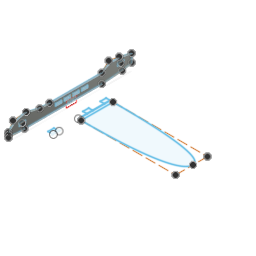
Plane v9 (Autodesk Fusion 360 design; units mm, degrees)
Autodesk Fusion 360 part; units mm, degrees
sketch "Body" plane through (0, 0, 0) normal (1, 0, 0) x (0, 0, -1)
  line L0 (-108.4233, 7.9987) -> (-100.7784, 21.612)
  line L1 (-100.7784, 21.612) -> (-77.9041, 23.072)
  spline S0 degree 2 poles (-108.4233, 7.9987) (-100.7784, 21.612) (-77.9041, 23.072) knots 0 0 0 1 1 1
  line L2 (-77.9041, 23.072) -> (-54.5916, 16.5393)
  line L3 (-54.5916, 16.5393) -> (-37.5103, 16.5393)
  spline S1 degree 2 poles (-77.9041, 23.072) (-54.5916, 16.5393) (-37.5103, 16.5393) knots 0 0 0 1 1 1
  line L4 (-37.5103, 16.5393) -> (52.5, 16.5392)
  line L5 (52.5, 16.5392) -> (64.5, 28.5)
  line L6 (64.5, 28.5) -> (82.5, 25.5)
  line L7 (82.5, 25.5) -> (104.0184, 19.9474)
  spline S2 degree 3 poles (52.5, 16.5392) (64.5, 28.5) (82.5, 25.5) (104.0184, 19.9474) knots 0 0 0 0 1 1 1 1
  line L8 (104.0184, 19.9474) -> (104.0184, 6)
  line L9 (104.0184, 6) -> (87.6259, 2.2265)
  line L10 (87.6259, 2.2265) -> (52.5, 0)
  spline S3 degree 2 poles (104.0184, 6) (87.6259, 2.2265) (52.5, 0) knots 0 0 0 1 1 1
  line L11 (52.5, 0) -> (-81.1435, 0.0002)
  line L12 (-108.4233, 7.9987) -> (-108.4233, 4.4987)
  line L13 (-108.4233, 4.4987) -> (-108.4233, -0.1059)
  line L14 (-108.4233, -0.1059) -> (-81.1435, 0.0002)
  spline S4 degree 2 poles (-108.4233, 4.4987) (-108.4233, -0.1059) (-81.1435, 0.0002) knots 0 0 0 1 1 1
  line L15 (0, 9) -> (2.5, 9) construction
  line L16 (2.5, 9) -> (2.5, 10.75) construction
  line L17 (2.5, 10.75) -> (12.5, 10.75)
  line L18 (12.5, 10.75) -> (12.5, 7.25)
  line L19 (12.5, 7.25) -> (2.5, 7.25)
  line L20 (2.5, 7.25) -> (2.5, 10.75)
  line L21 (12.5, 10.75) -> (17.5, 10.75) construction
  line L22 (17.5, 10.75) -> (27.5, 10.75)
  line L23 (27.5, 10.75) -> (27.5, 7.25)
  line L24 (27.5, 7.25) -> (17.5, 7.25)
  line L25 (17.5, 7.25) -> (17.5, 10.75)
  line L26 (0, 9) -> (-2.5, 9) construction
  line L27 (-2.5, 9) -> (-2.5, 10.75) construction
  line L28 (-2.5, 10.75) -> (-12.5, 10.75)
  line L29 (-12.5, 10.75) -> (-12.5, 7.25)
  line L30 (-12.5, 7.25) -> (-2.5, 7.25)
  line L31 (-2.5, 7.25) -> (-2.5, 10.75)
  line L32 (-12.5, 10.75) -> (-17.5, 10.75) construction
  line L33 (-17.5, 10.75) -> (-27.5, 10.75)
  line L34 (-27.5, 10.75) -> (-27.5, 7.25)
  line L35 (-27.5, 7.25) -> (-17.5, 7.25)
  line L36 (-17.5, 7.25) -> (-17.5, 10.75)
  line L37 (-80, 11.75) -> (-90, 11.75)
  line L38 (-90, 11.75) -> (-90, 8.25)
  line L39 (-90, 8.25) -> (-80, 8.25)
  line L40 (-80, 8.25) -> (-80, 11.75)
  line L41 (-80, 11.75) -> (-90, 8.25) construction
  line L42 (-90, 11.75) -> (-80, 8.25) construction
  line L43 (90, 13.25) -> (80, 13.25)
  line L44 (80, 13.25) -> (80, 16.75)
  line L45 (80, 16.75) -> (90, 16.75)
  line L46 (90, 16.75) -> (90, 13.25)
  line L47 (90, 13.25) -> (80, 16.75) construction
  line L48 (80, 13.25) -> (90, 16.75) construction
  point P0 (-85, 10)
  point P1 (85, 15)
  dimension "d5" = 3.5
  dimension "d69" = 2.5
  dimension "d70" = 1.75
  dimension "d71" = 10
  dimension "d72" = 3.5
  dimension "d73" = 5
  dimension "d74" = 10
  dimension "d75" = 3.5
  dimension "d76" = 2.5
  dimension "d77" = 1.75
  dimension "d78" = 10
  dimension "d79" = 3.5
  dimension "d80" = 5
  dimension "d81" = 10
  dimension "d82" = 3.5
  dimension "d94" = 10
  dimension "d95" = 3.5
  dimension "d102" = 10
  dimension "d103" = 3.5
  constraint vertical L8
  constraint parallel L4 L11
  constraint vertical L12
  constraint horizontal L15
  constraint perpendicular L15 L16
  constraint horizontal L17
  constraint vertical L18
  constraint horizontal L19
  constraint vertical L20
  constraint perpendicular L18 L21
  constraint horizontal L22
  constraint vertical L23
  constraint horizontal L24
  constraint vertical L25
  constraint parallel L15 L26
  constraint perpendicular L26 L27
  constraint horizontal L28
  constraint vertical L29
  constraint horizontal L30
  constraint vertical L31
  constraint perpendicular L29 L32
  constraint horizontal L33
  constraint vertical L34
  constraint horizontal L35
  constraint vertical L36
  constraint horizontal L37
  constraint perpendicular L37 L38
  constraint parallel L37 L39
  constraint parallel L38 L40
  constraint coincident L41 P0
  constraint coincident L42 P0
  constraint horizontal L43
  constraint perpendicular L43 L44
  constraint parallel L43 L45
  constraint parallel L44 L46
  constraint coincident L47 P1
  constraint coincident L48 P1
  measures "d5" distance of L0.start L12.end
  measures "d69" distance of L15.start L15.end
  measures "d70" distance of L15.end L16.end
  measures "d71" distance of L16.end L17.end
  measures "d72" distance of L16.end L19.end
  measures "d73" distance of L17.end L21.end
  measures "d74" distance of L21.end L22.end
  measures "d75" distance of L21.end L24.end
  measures "d76" distance of L15.start L26.end
  measures "d77" distance of L26.end L27.end
  measures "d78" distance of L27.end L28.end
  measures "d79" distance of L27.end L30.end
  measures "d80" distance of L28.end L32.end
  measures "d81" distance of L32.end L33.end
  measures "d82" distance of L32.end L35.end
  measures "d94" distance of L38.end L39.end
  measures "d95" distance of L37.end L38.end
  measures "d102" distance of L44.end L45.end
  measures "d103" distance of L43.end L44.end
sketch "Wing" plane through (0, 0, 0) normal (0, 1, 0) x (1, 0, 0)
  line L0 (25, 35) -> (32, 35)
  line L1 (32, 35) -> (32, 25)
  line L2 (32, 25) -> (25, 25)
  line L3 (25, 25) -> (25, 35)
  line L4 (32, 25) -> (32, 5)
  line L5 (32, 5) -> (25, 5)
  line L6 (25, 5) -> (25, -5)
  line L7 (25, -5) -> (32, -5)
  line L8 (32, -5) -> (32, 5)
  line L9 (32, -5) -> (32, -20)
  line L10 (32, 35) -> (37, 35)
  line L11 (37, 35) -> (37, -20)
  line L12 (37, -20) -> (32, -20)
  line L13 (32, -20) -> (32, 35)
  line L14 (37, 35) -> (200, 35)
  line L15 (200, 35) -> (200, 10)
  spline S0 degree 2 poles (37, 35) (200, 35) (200, 10) knots 0 0 0 1 1 1
  line L16 (37, -20) -> (200, -20)
  line L17 (200, -20) -> (200, 10)
  spline S1 degree 2 poles (37, -20) (200, -20) (200, 10) knots 0 0 0 1 1 1
  dimension "d84" = 7
  dimension "d85" = 10
  dimension "d86" = 20
  dimension "d87" = 7
  dimension "d88" = 10
  dimension "d89" = 15
  dimension "d90" = 5
  dimension "d91" = 55
  constraint horizontal L0
  constraint vertical L1
  constraint horizontal L2
  constraint vertical L3
  constraint perpendicular L2 L4
  constraint horizontal L5
  constraint vertical L6
  constraint horizontal L7
  constraint vertical L8
  constraint perpendicular L7 L9
  constraint horizontal L10
  constraint vertical L11
  constraint horizontal L12
  constraint vertical L13
  measures "d84" distance of L0.start L0.end
  measures "d85" distance of L0.start L2.end
  measures "d86" distance of L1.end L4.end
  measures "d87" distance of L4.end L5.end
  measures "d88" distance of L4.end L7.end
  measures "d89" distance of L7.end L9.end
  measures "d90" distance of L0.end L10.end
  measures "d91" distance of L0.end L9.end
sketch "Wedge" plane through (0, 0, 0) normal (0, 1, 0) x (1, 0, 0)
  line L0 (25, -55) -> (32, -55)
  line L1 (32, -55) -> (32, -65)
  line L2 (32, -65) -> (25, -65)
  line L3 (25, -65) -> (25, -55)
  line L4 (32, -55) -> (33.4142, -53.5858)
  line L5 (32, -55) -> (34, -55) construction
  line L6 (32, -65) -> (33.4142, -66.4142)
  line L7 (32, -65) -> (34, -65) construction
  line L8 (33.4142, -53.5858) -> (33.4142, -66.4142)
  dimension "d96" = 7
  dimension "d97" = 10
  dimension "d98" = 45
  dimension "d99" = 2
  dimension "d100" = 2
  dimension "d101" = 45
  constraint horizontal L0
  constraint vertical L1
  constraint horizontal L2
  constraint vertical L3
  constraint horizontal L5
  constraint horizontal L7
  measures "d96" distance of L0.start L0.end
  measures "d97" distance of L0.start L2.end
  measures "d98" angle of L4 L5
  measures "d99" distance of L0.end L4.end
  measures "d100" distance of L1.end L6.end
  measures "d101" angle of L6 L7
extrude "Extrude5" add sketch "Body" along normal blind 1 contours S0 L2 L3 L4 S2 L8 S3 L11 L12 S4 | L2 L3 S1 makes body 1
extrude "Extrude6" add sketch "Wing" along normal blind 1 separate body contours L0 L1 L2 L3 L13 | L1 L4 L8 L9 L10 L11 L12 L13 | L11 S0 S1 | L5 L6 L7 L8 L13 makes body 2
extrude "Extrude7" add sketch "Wedge" along normal blind 1 separate body makes body 3
extrude "Extrude8" add 1 faces at (33.4142, 0.3333, 57.8619) along direction (1, 0, 0) blind 1 on bodies 3 bodies 3
sketch "Connector" plane through (0, 0, 0) normal (0, 1, 0) x (1, 0, 0)
  line L0 (10, -40) -> (17, -40)
  line L1 (17, -40) -> (17, -45)
  line L2 (17, -45) -> (10, -45)
  line L3 (10, -45) -> (10, -40)
  dimension "d34" = 7
  dimension "d35" = 5
  constraint horizontal L0
  constraint vertical L1
  constraint horizontal L2
  constraint vertical L3
  measures "d34" distance of L0.start L0.end
  measures "d35" distance of L0.start L2.end
extrude "Extrude2" [suppressed]
extrude "Extrude3" [suppressed]
extrude "Extrude4" [suppressed]
hidden bodies 2 3
equation "width = 3.5 mm"
equation "d5 = width"
equation "d34 = width * 2"
equation "d70 = width / 2"
equation "d72 = width"
equation "d75 = width"
equation "d77 = width / 2"
equation "d79 = width"
equation "d82 = width"
equation "d84 = width * 2"
equation "d87 = width * 2"
equation "d95 = width"
equation "d96 = width * 2"
equation "d103 = width"
